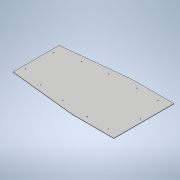
# Autodesk Inventor part: frontfloorfit2
Saved by Autodesk Inventor 2021 (Build 250183000, 183)
## iProperties
Created: 2020-10-26
Part Number: frontfloorfit2
Material: Generic
Document SubType Name: Modeling
Designer: mackeycj
Density: 1 g/cm^3
Appearance: Default
Author: mackeycj
Autodesk Inventor part; units mm, degrees
ref_plane "YZ Plane" through (0, 0, 0) normal (1, 0, 0) x (0, 1, 0)
ref_plane "XZ Plane" through (0, 0, 0) normal (0, 1, 0) x (-1, 0, 0)
ref_plane "XY Plane" through (0, 0, 0) normal (0, 0, 1) x (1, 0, 0)
sketch "Sketch1" plane through (0, 0, 0) normal (0, 1, 0) x (-1, 0, 0)
  line L0 (0, 0) -> (0, 215.9)
  line L1 (0, 215.9) -> (304.8, 215.9)
  line L2 (0, 0) -> (774.7, 0)
  line L3 (0, 0) -> (0, -215.9)
  line L4 (0, -215.9) -> (304.8, -215.9)
  line L5 (774.7, 0) -> (774.7, -165.1)
  line L6 (774.7, -165.1) -> (774.7, 0)
  line L7 (774.7, 0) -> (774.7, 165.1)
  line L8 (774.7, 165.1) -> (304.8, 215.9)
  line L9 (774.7, -165.1) -> (304.8, -215.9)
  line L10 (0, -215.9) -> (76.2, -215.9)
  line L11 (76.2, -215.9) -> (76.2, -177.8)
  line L12 (304.8, -215.9) -> (228.6, -215.9)
  line L13 (228.6, -215.9) -> (228.6, -177.8)
  line L14 (774.7, 0) -> (774.7, -101.6)
  line L15 (774.7, -101.6) -> (749.3, -101.6)
  line L16 (774.7, 0) -> (774.7, 101.6)
  line L17 (774.7, 101.6) -> (749.3, 101.6)
  line L18 (0, 215.9) -> (76.2, 215.9)
  line L19 (76.2, 215.9) -> (76.2, 177.8)
  line L20 (304.8, 215.9) -> (228.6, 215.9)
  line L21 (228.6, 215.9) -> (228.6, 177.8)
  line L22 (0, 0) -> (25.4, 0)
  line L23 (774.7, -165.1) -> (597.93, -184.2103)
  line L24 (597.93, -184.2103) -> (593.8349, -146.331)
  line L25 (597.93, -184.2103) -> (421.16, -203.3205)
  line L26 (421.16, -203.3205) -> (417.0649, -165.4413)
  line L27 (774.7, 165.1) -> (597.93, 184.2103)
  line L28 (597.93, 184.2103) -> (593.8349, 146.331)
  line L29 (597.93, 184.2103) -> (421.16, 203.3205)
  line L30 (421.16, 203.3205) -> (417.0649, 165.4413)
  dimension "d0" = 215.9
  dimension "d1" = 304.8
  dimension "d2" = 774.7
  dimension "d3" = 215.9
  dimension "d4" = 304.8
  dimension "d5" = 165.1
  dimension "d6" = 165.1
  dimension "d9" = 76.2
  dimension "d10" = 38.1
  dimension "d11" = 76.2
  dimension "d12" = 38.1
  dimension "d15" = 101.6
  dimension "d16" = 25.4
  dimension "d17" = 101.6
  dimension "d18" = 25.4
  dimension "d23" = 76.2
  dimension "d24" = 38.1
  dimension "d25" = 76.2
  dimension "d26" = 38.1
  dimension "d32" = 25.4
  dimension "d34" = 177.8
  dimension "d35" = 38.1
  dimension "d36" = 177.8
  dimension "d37" = 38.1
  dimension "d38" = 177.8
  dimension "d39" = 38.1
  dimension "d40" = 177.8
  dimension "d41" = 38.1
  constraints: 62 end point, 13 perpendicular, 11 point on line, 3 vertical, 1 collinear, 1 horizontal
  measures "d0" distance of L0.start L0.end
  measures "d1" distance of L0.end L1.end
  measures "d2" distance of L0.start L2.end
  measures "d3" distance of L0.start L3.end
  measures "d4" distance of L3.end L4.end
  measures "d5" distance of L2.end L5.end
  measures "d6" distance of L2.end L7.end
  measures "d9" distance of L3.end L10.end
  measures "d10" distance of L10.end L11.end
  measures "d11" distance of L4.end L12.end
  measures "d12" distance of L12.end L13.end
  measures "d15" distance of L2.end L14.end
  measures "d16" distance of L14.end L15.end
  measures "d17" distance of L2.end L16.end
  measures "d18" distance of L16.end L17.end
  measures "d23" distance of L0.end L18.end
  measures "d24" distance of L18.end L19.end
  measures "d25" distance of L1.end L20.end
  measures "d26" distance of L20.end L21.end
  measures "d32" distance of L0.start L22.end
  measures "d34" distance of L5.end L23.end
  measures "d35" distance of L23.end L24.end
  measures "d36" distance of L23.end L25.end
  measures "d37" distance of L25.end L26.end
  measures "d38" distance of L7.end L27.end
  measures "d39" distance of L27.end L28.end
  measures "d40" distance of L27.end L29.end
  measures "d41" distance of L29.end L30.end
extrude "Extrusion1" add sketch "Sketch1" along normal blind 3.175
hole "Hole1" at (-593.8349, 0, -146.331) at (-417.0649, 0, -165.4413) at (-228.6, 0, -177.8) at (-76.2, 0, -177.8) at (-76.2, 0, 177.8) at (-228.6, 0, 177.8) at (-417.0649, 0, 165.4413) at (-593.8349, 0, 146.331) at (-749.3, 0, 101.6) at (-749.3, 0, -101.6) at (-25.4, 0, 0) direction (0, 1, 0) diameter 5.1054 end through all clearance for "Flat Head Machine Screw (82)" size "#10" standard "Ansi Unified Screw Threads"
body "Solid1"
